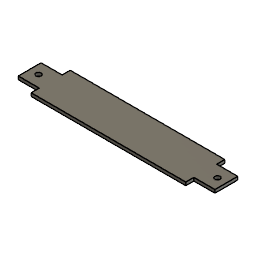
Tapa Pila (Autodesk Fusion 360 design; units mm, degrees)
part number: 2026-07-05-16-39-10-868
Autodesk Fusion 360 part; units mm, degrees
sketch "Boceto1" plane through (0, 0, 0) normal (0, 1, 0) x (1, 0, 0)
  line L0 (0, 0) -> (97.6, 0)
  line L1 (97.6, 0) -> (97.6, 26.186)
  line L2 (97.6, 26.186) -> (0, 26.186)
  line L3 (0, 26.186) -> (0, 0)
  dimension "d1" = 97.6
  dimension "d2" = 26.186
  constraint horizontal L0
  constraint vertical L1
  constraint horizontal L2
  constraint vertical L3
  constraint coincident L0.start L3.end
  measures "d1" distance of L0.start L0.end
  measures "d2" distance of L0.start L2.end
extrude "Extruir1" add sketch "Boceto1" along normal blind 2
sketch "Boceto2" plane through (0, 2, 0) normal (0, 1, 0) x (-1, 0, 0)
  line L0 (0, -26.186) -> (0, 0)
  line L1 (0, 0) -> (-97.6, 0)
  line L2 (-97.6, 0) -> (-97.6, -26.186)
  line L3 (-97.6, -26.186) -> (0, -26.186)
  line L4 (-97.6, -26.186) -> (-97.6, -13.093)
  line L5 (-97.6, -13.093) -> (-104.1, -13.093)
  circle A0 centre (-104.1, -13.093) radius 1.6
  line L6 (-97.6, -26.186) -> (-97.6, -21.186)
  line L7 (-97.6, -21.186) -> (-110.6, -21.186)
  line L8 (-110.6, -21.186) -> (-110.6, -5)
  line L9 (-110.6, -5) -> (-97.6, -5)
  line L10 (-97.6, -5) -> (-97.6, -21.186)
  dimension "d5" = 13.093
  dimension "d6" = 6.5
  dimension "d7" = 3.2
  dimension "d8" = 5
  dimension "d9" = 13
  dimension "d10" = 16.186
  constraint coincident L2.end L3.start
  constraint perpendicular L1 L4
  constraint perpendicular L4 L5
  constraint coincident L5.end A0.centre
  constraint perpendicular L3 L6
  constraint horizontal L7
  constraint vertical L8
  constraint horizontal L9
  constraint vertical L10
  measures "d5" distance of L2.end L4.end
  measures "d6" distance of L4.end L5.end
  measures "d7" diameter of A0
  measures "d8" distance of L2.end L6.end
  measures "d9" distance of L6.end L7.end
  measures "d10" distance of L6.end L9.end
extrude "Extruir2" add sketch "Boceto2" against normal blind 2 contours L2 L4 L7 L8 L9 L10
sketch "Boceto3" plane through (0, 2, 0) normal (0, 1, 0) x (-1, 0, 0)
  circle A0 centre (-104.1, -13.093) radius 1.6
  line L0 (0, -26.186) -> (0, 0)
  line L1 (0, 0) -> (-97.6, 0)
  line L2 (-97.6, 0) -> (-97.6, -5)
  line L3 (-97.6, -5) -> (-110.6, -5)
  line L4 (-110.6, -5) -> (-110.6, -21.186)
  line L5 (-110.6, -21.186) -> (-97.6, -21.186)
  line L6 (-97.6, -21.186) -> (-97.6, -26.186)
  line L7 (-97.6, -26.186) -> (0, -26.186)
  line L8 (0, -26.186) -> (0, -21.186)
  line L9 (0, -21.186) -> (13, -21.186)
  line L10 (13, -21.186) -> (13, -5)
  line L11 (13, -5) -> (0, -5)
  line L12 (0, -5) -> (0, -21.186)
  line L13 (0, -26.186) -> (0, -13.093)
  line L14 (0, -13.093) -> (6.5, -13.093)
  circle A1 centre (6.5, -13.093) radius 1.6
  dimension "d13" = 5
  dimension "d14" = 13
  dimension "d15" = 16.186
  dimension "d16" = 13.093
  dimension "d17" = 6.5
  dimension "d18" = 3.2
  constraint coincident L0.start L7.end
  constraint perpendicular L7 L8
  constraint horizontal L9
  constraint vertical L10
  constraint horizontal L11
  constraint vertical L12
  constraint perpendicular L1 L13
  constraint perpendicular L10 L14
  constraint coincident L14.end A1.centre
  measures "d13" distance of L0.start L8.end
  measures "d14" distance of L8.end L9.end
  measures "d15" distance of L8.end L11.end
  measures "d16" distance of L0.start L13.end
  measures "d17" distance of L13.end L14.end
  measures "d18" diameter of A1
extrude "Extruir3" add sketch "Boceto3" against normal blind 2 contours L0 L9 L10 L11 L12 L13
sketch "Boceto4" plane through (0, 2, 0) normal (0, 1, 0) x (-1, 0, 0)
  circle A0 centre (6.5, -13.093) radius 1.6
  circle A1 centre (-104.1, -13.093) radius 1.6
  line L0 (0, -26.186) -> (0, -21.186)
  line L1 (0, -21.186) -> (13, -21.186)
  line L2 (13, -21.186) -> (13, -5)
  line L3 (13, -5) -> (0, -5)
  line L4 (0, -5) -> (0, 0)
  line L5 (0, 0) -> (-97.6, 0)
  line L6 (-97.6, 0) -> (-97.6, -5)
  line L7 (-97.6, -5) -> (-110.6, -5)
  line L8 (-110.6, -5) -> (-110.6, -21.186)
  line L9 (-110.6, -21.186) -> (-97.6, -21.186)
  line L10 (-97.6, -21.186) -> (-97.6, -26.186)
  line L11 (-97.6, -26.186) -> (0, -26.186)
  line L12 (-96.6, -6) -> (-109.6, -6)
  line L13 (-109.6, -6) -> (-109.6, -20.186)
  line L14 (-109.6, -20.186) -> (-96.6, -20.186)
  line L15 (-96.6, -20.186) -> (-96.6, -25.186)
  line L16 (-96.6, -25.186) -> (-1, -25.186)
  line L17 (-1, -25.186) -> (-1, -20.186)
  line L18 (-1, -20.186) -> (12, -20.186)
  line L19 (12, -20.186) -> (12, -6)
  line L20 (12, -6) -> (-1, -6)
  line L21 (-1, -6) -> (-1, -1)
  line L22 (-1, -1) -> (-96.6, -1)
  line L23 (-96.6, -1) -> (-96.6, -6)
  dimension "d21" = -1
extrude "Extruir4" cut sketch "Boceto4" against normal blind 2 contours L0 L1 L2 L3 L4 L5 L6 L7 L8 L9 L10 L11
equation "d5 = 26.186 * 0.5 mm"
equation "d6 = ( 13 * 0.5 ) * 1 mm"
equation "d10 = 21.186 mm - 5 mm"
equation "d15 = 21.186 mm - 5 mm"
equation "d16 = 26.186 * 0.5 mm"
equation "d17 = 13.000 * 0.5 mm"
